Autodesk Fusion 360 part; units mm, degrees
note: some values were not read from the file. Chosen so that the rebuilt part matches the saved one: which bodies a step acts on. Set by a fixed rule: which sketch regions a step uses.
(part 2 of 2)
sketch "Sketch2" plane through (0, 0, 0) normal (0, 0, 1) x (1, 0, 0)
  line L0 (-3.5359, -0.6458) -> (-3.2779, -0.6913)
  line L1 (2.8438, -1.7707) -> (3.1017, -1.8162)
  arc A0 (3.1017, -1.8162) -> (3.681, -1.4106) centre (3.1886, -1.3238) ccw
  line L2 (3.681, -1.4106) -> (3.9414, 0.0666)
  arc A1 (3.9414, 0.0666) -> (3.5359, 0.6458) centre (3.449, 0.1534) ccw
  line L3 (3.5359, 0.6458) -> (3.2779, 0.6913)
  line L4 (-2.8438, 1.7707) -> (-3.1017, 1.8162)
  arc A2 (-3.1017, 1.8162) -> (-3.681, 1.4106) centre (-3.1886, 1.3238) ccw
  line L5 (-3.681, 1.4106) -> (-3.9414, -0.0666)
  arc A3 (-3.9414, -0.0666) -> (-3.5359, -0.6458) centre (-3.449, -0.1534) ccw
  line L6 (-1.7994, 9.2023) -> (-1.5414, 9.1568)
  line L7 (4.5803, 8.0774) -> (4.8382, 8.0319)
  arc A4 (4.8382, 8.0319) -> (5.4175, 8.4375) centre (4.925, 8.5243) ccw
  line L8 (5.4175, 8.4375) -> (5.6779, 9.9147)
  arc A5 (5.6779, 9.9147) -> (5.2723, 10.4939) centre (5.1855, 10.0015) ccw
  line L9 (5.2723, 10.4939) -> (5.0144, 10.5394)
  line L10 (-1.1073, 11.6188) -> (-1.3653, 11.6643)
  arc A6 (-1.3653, 11.6643) -> (-1.9445, 11.2587) centre (-1.4521, 11.1719) ccw
  line L11 (-1.9445, 11.2587) -> (-2.205, 9.7815)
  arc A7 (-2.205, 9.7815) -> (-1.7994, 9.2023) centre (-1.7126, 9.6947) ccw
  line L12 (-0.0629, 19.0503) -> (0.1951, 19.0049)
  line L13 (6.3167, 17.9254) -> (6.5747, 17.88)
  arc A8 (6.5747, 17.88) -> (7.1539, 18.2855) centre (6.6615, 18.3724) ccw
  line L14 (7.1539, 18.2855) -> (7.4144, 19.7627)
  arc A9 (7.4144, 19.7627) -> (7.0088, 20.342) centre (6.922, 19.8496) ccw
  line L15 (7.0088, 20.342) -> (6.7509, 20.3875)
  line L16 (0.6292, 21.4669) -> (0.3712, 21.5124)
  arc A10 (0.3712, 21.5124) -> (-0.208, 21.1068) centre (0.2844, 21.02) ccw
  line L17 (-0.208, 21.1068) -> (-0.4685, 19.6296)
  arc A11 (-0.4685, 19.6296) -> (-0.0629, 19.0503) centre (0.0239, 19.5427) ccw
  line L18 (1.6736, 28.8984) -> (1.9315, 28.8529)
  line L19 (8.0532, 27.7735) -> (8.3112, 27.728)
  arc A12 (8.3112, 27.728) -> (8.8904, 28.1336) centre (8.398, 28.2204) ccw
  line L20 (8.8904, 28.1336) -> (9.1509, 29.6108)
  arc A13 (9.1509, 29.6108) -> (8.7453, 30.19) centre (8.6585, 29.6976) ccw
  line L21 (8.7453, 30.19) -> (8.4873, 30.2355)
  line L22 (2.3657, 31.315) -> (2.1077, 31.3604)
  arc A14 (2.1077, 31.3604) -> (1.5285, 30.9549) centre (2.0209, 30.868) ccw
  line L23 (1.5285, 30.9549) -> (1.268, 29.4776)
  arc A15 (1.268, 29.4776) -> (1.6736, 28.8984) centre (1.7604, 29.3908) ccw
  line L24 (6.3122, -2.3823) -> (6.5702, -2.4278)
  line L25 (12.6919, -3.5072) -> (12.9498, -3.5527)
  arc A16 (12.9498, -3.5527) -> (13.529, -3.1471) centre (13.0366, -3.0603) ccw
  line L26 (13.529, -3.1471) -> (13.7895, -1.6699)
  arc A17 (13.7895, -1.6699) -> (13.3839, -1.0907) centre (13.2971, -1.5831) ccw
  line L27 (13.3839, -1.0907) -> (13.126, -1.0452)
  line L28 (7.0043, 0.0342) -> (6.7463, 0.0797)
  arc A18 (6.7463, 0.0797) -> (6.1671, -0.3259) centre (6.6595, -0.4127) ccw
  line L29 (6.1671, -0.3259) -> (5.9066, -1.8031)
  arc A19 (5.9066, -1.8031) -> (6.3122, -2.3823) centre (6.399, -1.8899) ccw
  line L30 (8.0487, 7.4658) -> (8.3067, 7.4203)
  line L31 (14.4283, 6.3409) -> (14.6863, 6.2954)
  arc A20 (14.6863, 6.2954) -> (15.2655, 6.701) centre (14.7731, 6.7878) ccw
  line L32 (15.2655, 6.701) -> (15.526, 8.1782)
  arc A21 (15.526, 8.1782) -> (15.1204, 8.7574) centre (15.0336, 8.265) ccw
  line L33 (15.1204, 8.7574) -> (14.8625, 8.8029)
  line L34 (8.7408, 9.8823) -> (8.4828, 9.9278)
  arc A22 (8.4828, 9.9278) -> (7.9036, 9.5222) centre (8.396, 9.4354) ccw
  line L35 (7.9036, 9.5222) -> (7.6431, 8.045)
  arc A23 (7.6431, 8.045) -> (8.0487, 7.4658) centre (8.1355, 7.9582) ccw
  line L36 (9.7852, 17.3139) -> (10.0431, 17.2684)
  line L37 (16.1648, 16.189) -> (16.4228, 16.1435)
  arc A24 (16.4228, 16.1435) -> (17.002, 16.549) centre (16.5096, 16.6359) ccw
  line L38 (17.002, 16.549) -> (17.2625, 18.0263)
  arc A25 (17.2625, 18.0263) -> (16.8569, 18.6055) centre (16.7701, 18.1131) ccw
  line L39 (16.8569, 18.6055) -> (16.5989, 18.651)
  line L40 (10.4773, 19.7304) -> (10.2193, 19.7759)
  arc A26 (10.2193, 19.7759) -> (9.6401, 19.3703) centre (10.1325, 19.2835) ccw
  line L41 (9.6401, 19.3703) -> (9.3796, 17.8931)
  arc A27 (9.3796, 17.8931) -> (9.7852, 17.3139) centre (9.872, 17.8063) ccw
  line L42 (11.5217, 27.1619) -> (11.7796, 27.1164)
  line L43 (17.9013, 26.037) -> (18.1593, 25.9915)
  arc A28 (18.1593, 25.9915) -> (18.7385, 26.3971) centre (18.2461, 26.484) ccw
  line L44 (18.7385, 26.3971) -> (18.999, 27.8743)
  arc A29 (18.999, 27.8743) -> (18.5934, 28.4536) centre (18.5066, 27.9612) ccw
  line L45 (18.5934, 28.4536) -> (18.3354, 28.4991)
  line L46 (12.2137, 29.5785) -> (11.9558, 29.624)
  arc A30 (11.9558, 29.624) -> (11.3766, 29.2184) centre (11.869, 29.1316) ccw
  line L47 (11.3766, 29.2184) -> (11.1161, 27.7412)
  arc A31 (11.1161, 27.7412) -> (11.5217, 27.1619) centre (11.6085, 27.6543) ccw
  line L48 (16.1603, -4.1188) -> (16.4183, -4.1643)
  line L49 (22.5399, -5.2437) -> (22.7979, -5.2892)
  arc A32 (22.7979, -5.2892) -> (23.3771, -4.8836) centre (22.8847, -4.7968) ccw
  line L50 (23.3771, -4.8836) -> (23.6376, -3.4064)
  arc A33 (23.6376, -3.4064) -> (23.232, -2.8271) centre (23.1452, -3.3196) ccw
  line L51 (23.232, -2.8271) -> (22.9741, -2.7817)
  line L52 (16.8524, -1.7022) -> (16.5944, -1.6568)
  arc A34 (16.5944, -1.6568) -> (16.0152, -2.0623) centre (16.5076, -2.1492) ccw
  line L53 (16.0152, -2.0623) -> (15.7547, -3.5396)
  arc A35 (15.7547, -3.5396) -> (16.1603, -4.1188) centre (16.2471, -3.6264) ccw
  line L54 (17.8968, 5.7293) -> (18.1547, 5.6838)
  line L55 (24.2764, 4.6044) -> (24.5344, 4.5589)
  arc A36 (24.5344, 4.5589) -> (25.1136, 4.9645) centre (24.6212, 5.0513) ccw
  line L56 (25.1136, 4.9645) -> (25.3741, 6.4417)
  arc A37 (25.3741, 6.4417) -> (24.9685, 7.0209) centre (24.8817, 6.5285) ccw
  line L57 (24.9685, 7.0209) -> (24.7105, 7.0664)
  line L58 (18.5889, 8.1458) -> (18.3309, 8.1913)
  arc A38 (18.3309, 8.1913) -> (17.7517, 7.7857) centre (18.2441, 7.6989) ccw
  line L59 (17.7517, 7.7857) -> (17.4912, 6.3085)
  arc A39 (17.4912, 6.3085) -> (17.8968, 5.7293) centre (17.9836, 6.2217) ccw
  line L60 (19.6333, 15.5774) -> (19.8912, 15.5319)
  line L61 (26.0129, 14.4525) -> (26.2709, 14.407)
  arc A40 (26.2709, 14.407) -> (26.8501, 14.8126) centre (26.3577, 14.8994) ccw
  line L62 (26.8501, 14.8126) -> (27.1106, 16.2898)
  arc A41 (27.1106, 16.2898) -> (26.705, 16.869) centre (26.6182, 16.3766) ccw
  line L63 (26.705, 16.869) -> (26.447, 16.9145)
  line L64 (20.3253, 17.9939) -> (20.0674, 18.0394)
  arc A42 (20.0674, 18.0394) -> (19.4881, 17.6338) centre (19.9806, 17.547) ccw
  line L65 (19.4881, 17.6338) -> (19.2277, 16.1566)
  arc A43 (19.2277, 16.1566) -> (19.6333, 15.5774) centre (19.7201, 16.0698) ccw
  line L66 (21.3697, 25.4255) -> (21.6277, 25.38)
  line L67 (27.7494, 24.3006) -> (28.0073, 24.2551)
  arc A44 (28.0073, 24.2551) -> (28.5866, 24.6606) centre (28.0942, 24.7475) ccw
  line L68 (28.5866, 24.6606) -> (28.847, 26.1379)
  arc A45 (28.847, 26.1379) -> (28.4415, 26.7171) centre (28.3546, 26.2247) ccw
  line L69 (28.4415, 26.7171) -> (28.1835, 26.7626)
  line L70 (22.0618, 27.842) -> (21.8039, 27.8875)
  arc A46 (21.8039, 27.8875) -> (21.2246, 27.4819) centre (21.717, 27.3951) ccw
  line L71 (21.2246, 27.4819) -> (20.9642, 26.0047)
  arc A47 (20.9642, 26.0047) -> (21.3697, 25.4255) centre (21.4566, 25.9179) ccw
  line L72 (26.0084, -5.8553) -> (26.2663, -5.9007)
  line L73 (32.388, -6.9802) -> (32.646, -7.0256)
  arc A48 (32.646, -7.0256) -> (33.2252, -6.6201) centre (32.7328, -6.5332) ccw
  line L74 (33.2252, -6.6201) -> (33.4857, -5.1429)
  arc A49 (33.4857, -5.1429) -> (33.0801, -4.5636) centre (32.9933, -5.056) ccw
  line L75 (33.0801, -4.5636) -> (32.8221, -4.5181)
  line L76 (26.7005, -3.4387) -> (26.4425, -3.3932)
  arc A50 (26.4425, -3.3932) -> (25.8633, -3.7988) centre (26.3557, -3.8856) ccw
  line L77 (25.8633, -3.7988) -> (25.6028, -5.276)
  arc A51 (25.6028, -5.276) -> (26.0084, -5.8553) centre (26.0952, -5.3629) ccw
  line L78 (27.7449, 3.9928) -> (28.0028, 3.9473)
  line L79 (34.1245, 2.8679) -> (34.3825, 2.8224)
  arc A52 (34.3825, 2.8224) -> (34.9617, 3.228) centre (34.4693, 3.3148) ccw
  line L80 (34.9617, 3.228) -> (35.2222, 4.7052)
  arc A53 (35.2222, 4.7052) -> (34.8166, 5.2844) centre (34.7298, 4.792) ccw
  line L81 (34.8166, 5.2844) -> (34.5586, 5.3299)
  line L82 (28.4369, 6.4093) -> (28.179, 6.4548)
  arc A54 (28.179, 6.4548) -> (27.5997, 6.0493) centre (28.0921, 5.9624) ccw
  line L83 (27.5997, 6.0493) -> (27.3393, 4.572)
  arc A55 (27.3393, 4.572) -> (27.7449, 3.9928) centre (27.8317, 4.4852) ccw
  line L84 (29.4813, 13.8409) -> (29.7393, 13.7954)
  line L85 (35.861, 12.716) -> (36.1189, 12.6705)
  arc A56 (36.1189, 12.6705) -> (36.6982, 13.0761) centre (36.2058, 13.1629) ccw
  line L86 (36.6982, 13.0761) -> (36.9586, 14.5533)
  arc A57 (36.9586, 14.5533) -> (36.5531, 15.1325) centre (36.4662, 14.6401) ccw
  line L87 (36.5531, 15.1325) -> (36.2951, 15.178)
  line L88 (30.1734, 16.2574) -> (29.9155, 16.3029)
  arc A58 (29.9155, 16.3029) -> (29.3362, 15.8973) centre (29.8286, 15.8105) ccw
  line L89 (29.3362, 15.8973) -> (29.0758, 14.4201)
  arc A59 (29.0758, 14.4201) -> (29.4813, 13.8409) centre (29.5682, 14.3333) ccw
  line L90 (31.2178, 23.689) -> (31.4758, 23.6435)
  line L91 (37.5975, 22.5641) -> (37.8554, 22.5186)
  arc A60 (37.8554, 22.5186) -> (38.4346, 22.9242) centre (37.9422, 23.011) ccw
  line L92 (38.4346, 22.9242) -> (38.6951, 24.4014)
  arc A61 (38.6951, 24.4014) -> (38.2895, 24.9806) centre (38.2027, 24.4882) ccw
  line L93 (38.2895, 24.9806) -> (38.0316, 25.0261)
  line L94 (31.9099, 26.1055) -> (31.6519, 26.151)
  arc A62 (31.6519, 26.151) -> (31.0727, 25.7454) centre (31.5651, 25.6586) ccw
  line L95 (31.0727, 25.7454) -> (30.8122, 24.2682)
  arc A63 (30.8122, 24.2682) -> (31.2178, 23.689) centre (31.3046, 24.1814) ccw
  line L96 (35.8564, -7.5917) -> (36.1144, -7.6372)
  line L97 (42.2361, -8.7166) -> (42.4941, -8.7621)
  arc A64 (42.4941, -8.7621) -> (43.0733, -8.3566) centre (42.5809, -8.2697) ccw
  line L98 (43.0733, -8.3566) -> (43.3338, -6.8793)
  arc A65 (43.3338, -6.8793) -> (42.9282, -6.3001) centre (42.8413, -6.7925) ccw
  line L99 (42.9282, -6.3001) -> (42.6702, -6.2546)
  line L100 (36.5485, -5.1752) -> (36.2906, -5.1297)
  arc A66 (36.2906, -5.1297) -> (35.7113, -5.5353) centre (36.2037, -5.6221) ccw
  line L101 (35.7113, -5.5353) -> (35.4509, -7.0125)
  arc A67 (35.4509, -7.0125) -> (35.8564, -7.5917) centre (35.9433, -7.0993) ccw
  line L102 (37.5929, 2.2563) -> (37.8509, 2.2108)
  line L103 (43.9726, 1.1314) -> (44.2305, 1.0859)
  arc A68 (44.2305, 1.0859) -> (44.8098, 1.4915) centre (44.3174, 1.5784) ccw
  line L104 (44.8098, 1.4915) -> (45.0702, 2.9687)
  arc A69 (45.0702, 2.9687) -> (44.6647, 3.548) centre (44.5778, 3.0556) ccw
  line L105 (44.6647, 3.548) -> (44.4067, 3.5935)
  line L106 (38.285, 4.6729) -> (38.0271, 4.7184)
  arc A70 (38.0271, 4.7184) -> (37.4478, 4.3128) centre (37.9402, 4.226) ccw
  line L107 (37.4478, 4.3128) -> (37.1873, 2.8356)
  arc A71 (37.1873, 2.8356) -> (37.5929, 2.2563) centre (37.6798, 2.7487) ccw
  line L108 (39.3294, 12.1044) -> (39.5874, 12.0589)
  line L109 (45.709, 10.9795) -> (45.967, 10.934)
  arc A72 (45.967, 10.934) -> (46.5462, 11.3396) centre (46.0538, 11.4264) ccw
  line L110 (46.5462, 11.3396) -> (46.8067, 12.8168)
  arc A73 (46.8067, 12.8168) -> (46.4011, 13.396) centre (46.3143, 12.9036) ccw
  line L111 (46.4011, 13.396) -> (46.1432, 13.4415)
  line L112 (40.0215, 14.5209) -> (39.7635, 14.5664)
  arc A74 (39.7635, 14.5664) -> (39.1843, 14.1609) centre (39.6767, 14.074) ccw
  line L113 (39.1843, 14.1609) -> (38.9238, 12.6836)
  arc A75 (38.9238, 12.6836) -> (39.3294, 12.1044) centre (39.4162, 12.5968) ccw
  line L114 (41.0659, 21.9525) -> (41.3239, 21.907)
  line L115 (47.4455, 20.8276) -> (47.7035, 20.7821)
  arc A76 (47.7035, 20.7821) -> (48.2827, 21.1877) centre (47.7903, 21.2745) ccw
  line L116 (48.2827, 21.1877) -> (48.5432, 22.6649)
  arc A77 (48.5432, 22.6649) -> (48.1376, 23.2441) centre (48.0508, 22.7517) ccw
  line L117 (48.1376, 23.2441) -> (47.8797, 23.2896)
  line L118 (41.758, 24.369) -> (41.5, 24.4145)
  arc A78 (41.5, 24.4145) -> (40.9208, 24.0089) centre (41.4132, 23.9221) ccw
  line L119 (40.9208, 24.0089) -> (40.6603, 22.5317)
  arc A79 (40.6603, 22.5317) -> (41.0659, 21.9525) centre (41.1527, 22.4449) ccw
  line L120 (101.6288, -1.8162) -> (101.8868, -1.7707)
  line L121 (108.0084, -0.6913) -> (108.2664, -0.6458)
  arc A80 (108.2664, -0.6458) -> (108.672, -0.0666) centre (108.1796, -0.1534) ccw
  line L122 (108.672, -0.0666) -> (108.4115, 1.4106)
  arc A81 (108.4115, 1.4106) -> (107.8323, 1.8162) centre (107.9191, 1.3238) ccw
  line L123 (107.8323, 1.8162) -> (107.5743, 1.7707)
  line L124 (101.4527, 0.6913) -> (101.1947, 0.6458)
  arc A82 (101.1947, 0.6458) -> (100.7891, 0.0666) centre (101.2815, 0.1534) ccw
  line L125 (100.7891, 0.0666) -> (101.0496, -1.4106)
  arc A83 (101.0496, -1.4106) -> (101.6288, -1.8162) centre (101.542, -1.3238) ccw
  line L126 (99.8923, 8.0319) -> (100.1503, 8.0774)
  line L127 (106.272, 9.1568) -> (106.5299, 9.2023)
  arc A84 (106.5299, 9.2023) -> (106.9355, 9.7815) centre (106.4431, 9.6947) ccw
  line L128 (106.9355, 9.7815) -> (106.675, 11.2587)
  arc A85 (106.675, 11.2587) -> (106.0958, 11.6643) centre (106.1826, 11.1719) ccw
  line L129 (106.0958, 11.6643) -> (105.8378, 11.6188)
  line L130 (99.7162, 10.5394) -> (99.4582, 10.4939)
  arc A86 (99.4582, 10.4939) -> (99.0526, 9.9147) centre (99.545, 10.0015) ccw
  line L131 (99.0526, 9.9147) -> (99.3131, 8.4375)
  arc A87 (99.3131, 8.4375) -> (99.8923, 8.0319) centre (99.8055, 8.5243) ccw
  line L132 (98.1558, 17.88) -> (98.4138, 17.9254)
  line L133 (104.5355, 19.0049) -> (104.7934, 19.0503)
  arc A88 (104.7934, 19.0503) -> (105.199, 19.6296) centre (104.7066, 19.5427) ccw
  line L134 (105.199, 19.6296) -> (104.9386, 21.1068)
  arc A89 (104.9386, 21.1068) -> (104.3593, 21.5124) centre (104.4461, 21.02) ccw
  line L135 (104.3593, 21.5124) -> (104.1014, 21.4669)
  line L136 (97.9797, 20.3875) -> (97.7217, 20.342)
  arc A90 (97.7217, 20.342) -> (97.3161, 19.7627) centre (97.8085, 19.8496) ccw
  line L137 (97.3161, 19.7627) -> (97.5766, 18.2855)
  arc A91 (97.5766, 18.2855) -> (98.1558, 17.88) centre (98.069, 18.3724) ccw
  line L138 (96.4194, 27.728) -> (96.6773, 27.7735)
  line L139 (102.799, 28.8529) -> (103.057, 28.8984)
  arc A92 (103.057, 28.8984) -> (103.4625, 29.4776) centre (102.9701, 29.3908) ccw
  line L140 (103.4625, 29.4776) -> (103.2021, 30.9549)
  arc A93 (103.2021, 30.9549) -> (102.6228, 31.3604) centre (102.7097, 30.868) ccw
  line L141 (102.6228, 31.3604) -> (102.3649, 31.315)
  line L142 (96.2432, 30.2355) -> (95.9852, 30.19)
  arc A94 (95.9852, 30.19) -> (95.5797, 29.6108) centre (96.0721, 29.6976) ccw
  line L143 (95.5797, 29.6108) -> (95.8401, 28.1336)
  arc A95 (95.8401, 28.1336) -> (96.4194, 27.728) centre (96.3325, 28.2204) ccw
  line L144 (91.7807, -3.5527) -> (92.0387, -3.5072)
  line L145 (98.1604, -2.4278) -> (98.4183, -2.3823)
  arc A96 (98.4183, -2.3823) -> (98.8239, -1.8031) centre (98.3315, -1.8899) ccw
  line L146 (98.8239, -1.8031) -> (98.5634, -0.3259)
  arc A97 (98.5634, -0.3259) -> (97.9842, 0.0797) centre (98.071, -0.4127) ccw
  line L147 (97.9842, 0.0797) -> (97.7262, 0.0342)
  line L148 (91.6046, -1.0452) -> (91.3466, -1.0907)
  arc A98 (91.3466, -1.0907) -> (90.941, -1.6699) centre (91.4334, -1.5831) ccw
  line L149 (90.941, -1.6699) -> (91.2015, -3.1471)
  arc A99 (91.2015, -3.1471) -> (91.7807, -3.5527) centre (91.6939, -3.0603) ccw
  line L150 (90.0442, 6.2954) -> (90.3022, 6.3409)
  line L151 (96.4239, 7.4203) -> (96.6819, 7.4658)
  arc A100 (96.6819, 7.4658) -> (97.0874, 8.045) centre (96.595, 7.9582) ccw
  line L152 (97.0874, 8.045) -> (96.827, 9.5222)
  arc A101 (96.827, 9.5222) -> (96.2477, 9.9278) centre (96.3346, 9.4354) ccw
  line L153 (96.2477, 9.9278) -> (95.9898, 9.8823)
  line L154 (89.8681, 8.8029) -> (89.6101, 8.7574)
  arc A102 (89.6101, 8.7574) -> (89.2045, 8.1782) centre (89.6969, 8.265) ccw
  line L155 (89.2045, 8.1782) -> (89.465, 6.701)
  arc A103 (89.465, 6.701) -> (90.0442, 6.2954) centre (89.9574, 6.7878) ccw
  line L156 (88.3078, 16.1435) -> (88.5657, 16.189)
  line L157 (94.6874, 17.2684) -> (94.9454, 17.3139)
  arc A104 (94.9454, 17.3139) -> (95.3509, 17.8931) centre (94.8585, 17.8063) ccw
  line L158 (95.3509, 17.8931) -> (95.0905, 19.3703)
  arc A105 (95.0905, 19.3703) -> (94.5112, 19.7759) centre (94.5981, 19.2835) ccw
  line L159 (94.5112, 19.7759) -> (94.2533, 19.7304)
  line L160 (88.1316, 18.651) -> (87.8736, 18.6055)
  arc A106 (87.8736, 18.6055) -> (87.4681, 18.0263) centre (87.9605, 18.1131) ccw
  line L161 (87.4681, 18.0263) -> (87.7285, 16.549)
  arc A107 (87.7285, 16.549) -> (88.3078, 16.1435) centre (88.2209, 16.6359) ccw
  line L162 (86.5713, 25.9915) -> (86.8292, 26.037)
  line L163 (92.9509, 27.1164) -> (93.2089, 27.1619)
  arc A108 (93.2089, 27.1619) -> (93.6145, 27.7412) centre (93.1221, 27.6543) ccw
  line L164 (93.6145, 27.7412) -> (93.354, 29.2184)
  arc A109 (93.354, 29.2184) -> (92.7748, 29.624) centre (92.8616, 29.1316) ccw
  line L165 (92.7748, 29.624) -> (92.5168, 29.5785)
  line L166 (86.3951, 28.4991) -> (86.1372, 28.4536)
  arc A110 (86.1372, 28.4536) -> (85.7316, 27.8743) centre (86.224, 27.9612) ccw
  line L167 (85.7316, 27.8743) -> (85.9921, 26.3971)
  arc A111 (85.9921, 26.3971) -> (86.5713, 25.9915) centre (86.4845, 26.484) ccw
  line L168 (81.9327, -5.2892) -> (82.1906, -5.2437)
  line L169 (88.3123, -4.1643) -> (88.5703, -4.1188)
  arc A112 (88.5703, -4.1188) -> (88.9758, -3.5396) centre (88.4834, -3.6264) ccw
  line L170 (88.9758, -3.5396) -> (88.7154, -2.0623)
  arc A113 (88.7154, -2.0623) -> (88.1361, -1.6568) centre (88.223, -2.1492) ccw
  line L171 (88.1361, -1.6568) -> (87.8782, -1.7022)
  line L172 (81.7565, -2.7817) -> (81.4985, -2.8271)
  arc A114 (81.4985, -2.8271) -> (81.093, -3.4064) centre (81.5854, -3.3196) ccw
  line L173 (81.093, -3.4064) -> (81.3534, -4.8836)
  arc A115 (81.3534, -4.8836) -> (81.9327, -5.2892) centre (81.8458, -4.7968) ccw
  line L174 (80.1962, 4.5589) -> (80.4541, 4.6044)
  line L175 (86.5758, 5.6838) -> (86.8338, 5.7293)
  arc A116 (86.8338, 5.7293) -> (87.2394, 6.3085) centre (86.7469, 6.2217) ccw
  line L176 (87.2394, 6.3085) -> (86.9789, 7.7857)
  arc A117 (86.9789, 7.7857) -> (86.3997, 8.1913) centre (86.4865, 7.6989) ccw
  line L177 (86.3997, 8.1913) -> (86.1417, 8.1458)
  line L178 (80.02, 7.0664) -> (79.762, 7.0209)
  arc A118 (79.762, 7.0209) -> (79.3565, 6.4417) centre (79.8489, 6.5285) ccw
  line L179 (79.3565, 6.4417) -> (79.6169, 4.9645)
  arc A119 (79.6169, 4.9645) -> (80.1962, 4.5589) centre (80.1093, 5.0513) ccw
  line L180 (78.4597, 14.407) -> (78.7177, 14.4525)
  line L181 (84.8393, 15.5319) -> (85.0973, 15.5774)
  arc A120 (85.0973, 15.5774) -> (85.5029, 16.1566) centre (85.0105, 16.0698) ccw
  line L182 (85.5029, 16.1566) -> (85.2424, 17.6338)
  arc A121 (85.2424, 17.6338) -> (84.6632, 18.0394) centre (84.75, 17.547) ccw
  line L183 (84.6632, 18.0394) -> (84.4052, 17.9939)
  line L184 (78.2835, 16.9145) -> (78.0256, 16.869)
  arc A122 (78.0256, 16.869) -> (77.62, 16.2898) centre (78.1124, 16.3766) ccw
  line L185 (77.62, 16.2898) -> (77.8805, 14.8126)
  arc A123 (77.8805, 14.8126) -> (78.4597, 14.407) centre (78.3729, 14.8994) ccw
  line L186 (76.7232, 24.2551) -> (76.9812, 24.3006)
  line L187 (83.1028, 25.38) -> (83.3608, 25.4255)
  arc A124 (83.3608, 25.4255) -> (83.7664, 26.0047) centre (83.274, 25.9179) ccw
  line L188 (83.7664, 26.0047) -> (83.5059, 27.4819)
  arc A125 (83.5059, 27.4819) -> (82.9267, 27.8875) centre (83.0135, 27.3951) ccw
  line L189 (82.9267, 27.8875) -> (82.6687, 27.842)
  line L190 (76.5471, 26.7626) -> (76.2891, 26.7171)
  arc A126 (76.2891, 26.7171) -> (75.8835, 26.1379) centre (76.3759, 26.2247) ccw
  line L191 (75.8835, 26.1379) -> (76.144, 24.6606)
  arc A127 (76.144, 24.6606) -> (76.7232, 24.2551) centre (76.6364, 24.7475) ccw
  line L192 (72.0846, -7.0256) -> (72.3425, -6.9802)
  line L193 (78.4642, -5.9007) -> (78.7222, -5.8553)
  arc A128 (78.7222, -5.8553) -> (79.1278, -5.276) centre (78.6354, -5.3629) ccw
  line L194 (79.1278, -5.276) -> (78.8673, -3.7988)
  arc A129 (78.8673, -3.7988) -> (78.2881, -3.3932) centre (78.3749, -3.8856) ccw
  line L195 (78.2881, -3.3932) -> (78.0301, -3.4387)
  line L196 (71.9084, -4.5181) -> (71.6505, -4.5636)
  arc A130 (71.6505, -4.5636) -> (71.2449, -5.1429) centre (71.7373, -5.056) ccw
  line L197 (71.2449, -5.1429) -> (71.5053, -6.6201)
  arc A131 (71.5053, -6.6201) -> (72.0846, -7.0256) centre (71.9977, -6.5332) ccw
  line L198 (70.3481, 2.8224) -> (70.6061, 2.8679)
  line L199 (76.7277, 3.9473) -> (76.9857, 3.9928)
  arc A132 (76.9857, 3.9928) -> (77.3913, 4.572) centre (76.8989, 4.4852) ccw
  line L200 (77.3913, 4.572) -> (77.1308, 6.0493)
  arc A133 (77.1308, 6.0493) -> (76.5516, 6.4548) centre (76.6384, 5.9624) ccw
  line L201 (76.5516, 6.4548) -> (76.2936, 6.4093)
  line L202 (70.1719, 5.3299) -> (69.914, 5.2844)
  arc A134 (69.914, 5.2844) -> (69.5084, 4.7052) centre (70.0008, 4.792) ccw
  line L203 (69.5084, 4.7052) -> (69.7689, 3.228)
  arc A135 (69.7689, 3.228) -> (70.3481, 2.8224) centre (70.2613, 3.3148) ccw
  line L204 (68.6116, 12.6705) -> (68.8696, 12.716)
  line L205 (74.9912, 13.7954) -> (75.2492, 13.8409)
  arc A136 (75.2492, 13.8409) -> (75.6548, 14.4201) centre (75.1624, 14.3333) ccw
  line L206 (75.6548, 14.4201) -> (75.3943, 15.8973)
  arc A137 (75.3943, 15.8973) -> (74.8151, 16.3029) centre (74.9019, 15.8105) ccw
  line L207 (74.8151, 16.3029) -> (74.5571, 16.2574)
  line L208 (68.4355, 15.178) -> (68.1775, 15.1325)
  arc A138 (68.1775, 15.1325) -> (67.7719, 14.5533) centre (68.2643, 14.6401) ccw
  line L209 (67.7719, 14.5533) -> (68.0324, 13.0761)
  arc A139 (68.0324, 13.0761) -> (68.6116, 12.6705) centre (68.5248, 13.1629) ccw
  line L210 (66.8751, 22.5186) -> (67.1331, 22.5641)
  line L211 (73.2548, 23.6435) -> (73.5127, 23.689)
  arc A140 (73.5127, 23.689) -> (73.9183, 24.2682) centre (73.4259, 24.1814) ccw
  line L212 (73.9183, 24.2682) -> (73.6578, 25.7454)
  arc A141 (73.6578, 25.7454) -> (73.0786, 26.151) centre (73.1654, 25.6586) ccw
  line L213 (73.0786, 26.151) -> (72.8206, 26.1055)
  line L214 (66.699, 25.0261) -> (66.441, 24.9806)
  arc A142 (66.441, 24.9806) -> (66.0354, 24.4014) centre (66.5278, 24.4882) ccw
  line L215 (66.0354, 24.4014) -> (66.2959, 22.9242)
  arc A143 (66.2959, 22.9242) -> (66.8751, 22.5186) centre (66.7883, 23.011) ccw
  line L216 (62.2365, -8.7621) -> (62.4945, -8.7166)
  line L217 (68.6161, -7.6372) -> (68.8741, -7.5917)
  arc A144 (68.8741, -7.5917) -> (69.2797, -7.0125) centre (68.7873, -7.0993) ccw
  line L218 (69.2797, -7.0125) -> (69.0192, -5.5353)
  arc A145 (69.0192, -5.5353) -> (68.44, -5.1297) centre (68.5268, -5.6221) ccw
  line L219 (68.44, -5.1297) -> (68.182, -5.1752)
  line L220 (62.0603, -6.2546) -> (61.8024, -6.3001)
  arc A146 (61.8024, -6.3001) -> (61.3968, -6.8793) centre (61.8892, -6.7925) ccw
  line L221 (61.3968, -6.8793) -> (61.6573, -8.3566)
  arc A147 (61.6573, -8.3566) -> (62.2365, -8.7621) centre (62.1497, -8.2697) ccw
  line L222 (60.5, 1.0859) -> (60.758, 1.1314)
  line L223 (66.8797, 2.2108) -> (67.1376, 2.2563)
  arc A148 (67.1376, 2.2563) -> (67.5432, 2.8356) centre (67.0508, 2.7487) ccw
  line L224 (67.5432, 2.8356) -> (67.2827, 4.3128)
  arc A149 (67.2827, 4.3128) -> (66.7035, 4.7184) centre (66.7903, 4.226) ccw
  line L225 (66.7035, 4.7184) -> (66.4455, 4.6729)
  line L226 (60.3239, 3.5935) -> (60.0659, 3.548)
  arc A150 (60.0659, 3.548) -> (59.6603, 2.9687) centre (60.1527, 3.0556) ccw
  line L227 (59.6603, 2.9687) -> (59.9208, 1.4915)
  arc A151 (59.9208, 1.4915) -> (60.5, 1.0859) centre (60.4132, 1.5784) ccw
  line L228 (58.7635, 10.934) -> (59.0215, 10.9795)
  line L229 (65.1432, 12.0589) -> (65.4011, 12.1044)
  arc A152 (65.4011, 12.1044) -> (65.8067, 12.6836) centre (65.3143, 12.5968) ccw
  line L230 (65.8067, 12.6836) -> (65.5462, 14.1609)
  arc A153 (65.5462, 14.1609) -> (64.967, 14.5664) centre (65.0538, 14.074) ccw
  line L231 (64.967, 14.5664) -> (64.709, 14.5209)
  line L232 (58.5874, 13.4415) -> (58.3294, 13.396)
  arc A154 (58.3294, 13.396) -> (57.9238, 12.8168) centre (58.4162, 12.9036) ccw
  line L233 (57.9238, 12.8168) -> (58.1843, 11.3396)
  arc A155 (58.1843, 11.3396) -> (58.7635, 10.934) centre (58.6767, 11.4264) ccw
  line L234 (57.0271, 20.7821) -> (57.285, 20.8276)
  line L235 (63.4067, 21.907) -> (63.6647, 21.9525)
  arc A156 (63.6647, 21.9525) -> (64.0702, 22.5317) centre (63.5778, 22.4449) ccw
  line L236 (64.0702, 22.5317) -> (63.8098, 24.0089)
  arc A157 (63.8098, 24.0089) -> (63.2305, 24.4145) centre (63.3174, 23.9221) ccw
  line L237 (63.2305, 24.4145) -> (62.9726, 24.369)
  line L238 (56.8509, 23.2896) -> (56.5929, 23.2441)
  arc A158 (56.5929, 23.2441) -> (56.1873, 22.6649) centre (56.6798, 22.7517) ccw
  line L239 (56.1873, 22.6649) -> (56.4478, 21.1877)
  arc A159 (56.4478, 21.1877) -> (57.0271, 20.7821) centre (56.9402, 21.2745) ccw
  arc A160 (-3.2779, -0.6913) -> (-3.2779, -0.6913) centre (0, 0) ccw
  arc A161 (-1.5414, 9.1568) -> (-1.5414, 9.1568) centre (1.7365, 9.8481) ccw
  arc A162 (0.1951, 19.0049) -> (0.1951, 19.0049) centre (3.473, 19.6962) ccw
  arc A163 (1.9315, 28.8529) -> (1.9315, 28.8529) centre (5.2094, 29.5442) ccw
  arc A164 (6.5702, -2.4278) -> (6.5702, -2.4278) centre (9.8481, -1.7365) ccw
  arc A165 (8.3067, 7.4203) -> (8.3067, 7.4203) centre (11.5846, 8.1116) ccw
  arc A166 (10.0431, 17.2684) -> (10.0431, 17.2684) centre (13.321, 17.9597) ccw
  arc A167 (11.7796, 27.1164) -> (11.7796, 27.1164) centre (15.0575, 27.8078) ccw
  arc A168 (16.4183, -4.1643) -> (16.4183, -4.1643) centre (19.6962, -3.473) ccw
  arc A169 (18.1547, 5.6838) -> (18.1547, 5.6838) centre (21.4326, 6.3751) ccw
  arc A170 (19.8912, 15.5319) -> (19.8912, 15.5319) centre (23.1691, 16.2232) ccw
  arc A171 (21.6277, 25.38) -> (21.6277, 25.38) centre (24.9056, 26.0713) ccw
  arc A172 (26.2663, -5.9007) -> (26.2663, -5.9007) centre (29.5442, -5.2094) ccw
  arc A173 (28.0028, 3.9473) -> (28.0028, 3.9473) centre (31.2807, 4.6386) ccw
  arc A174 (29.7393, 13.7954) -> (29.7393, 13.7954) centre (33.0172, 14.4867) ccw
  arc A175 (31.4758, 23.6435) -> (31.4758, 23.6435) centre (34.7537, 24.3348) ccw
  arc A176 (36.1144, -7.6372) -> (36.1144, -7.6372) centre (39.3923, -6.9459) ccw
  arc A177 (37.8509, 2.2108) -> (37.8509, 2.2108) centre (41.1288, 2.9022) ccw
  arc A178 (39.5874, 12.0589) -> (39.5874, 12.0589) centre (42.8653, 12.7502) ccw
  arc A179 (41.3239, 21.907) -> (41.3239, 21.907) centre (44.6018, 22.5983) ccw
  circle A180 centre (104.7305, 0) radius 3.35
  circle A181 centre (102.9941, 9.8481) radius 3.35
  circle A182 centre (101.2576, 19.6962) radius 3.35
  circle A183 centre (99.5211, 29.5442) radius 3.35
  circle A184 centre (94.8825, -1.7365) radius 3.35
  circle A185 centre (93.146, 8.1116) radius 3.35
  circle A186 centre (91.4095, 17.9597) radius 3.35
  circle A187 centre (89.673, 27.8078) radius 3.35
  circle A188 centre (85.0344, -3.473) radius 3.35
  circle A189 centre (83.2979, 6.3751) radius 3.35
  circle A190 centre (81.5614, 16.2232) radius 3.35
  circle A191 centre (79.8249, 26.0713) radius 3.35
  circle A192 centre (75.1863, -5.2094) radius 3.35
  circle A193 centre (73.4498, 4.6386) radius 3.35
  circle A194 centre (71.7134, 14.4867) radius 3.35
  circle A195 centre (69.9769, 24.3348) radius 3.35
  circle A196 centre (65.3382, -6.9459) radius 3.35
  circle A197 centre (63.6018, 2.9022) radius 3.35
  circle A198 centre (61.8653, 12.7502) radius 3.35
  circle A199 centre (60.1288, 22.5983) radius 3.35
  circle A200 centre (5.2094, 29.5442) radius 3.35
  circle A201 centre (15.0575, 27.8078) radius 3.35
  circle A202 centre (24.9056, 26.0713) radius 3.35
  circle A203 centre (34.7537, 24.3348) radius 3.35
  circle A204 centre (44.6018, 22.5983) radius 3.35
  circle A205 centre (42.8653, 12.7502) radius 3.35
  circle A206 centre (33.0172, 14.4867) radius 3.35
  circle A207 centre (23.1691, 16.2232) radius 3.35
  circle A208 centre (13.321, 17.9597) radius 3.35
  circle A209 centre (3.473, 19.6962) radius 3.35
  circle A210 centre (1.7365, 9.8481) radius 3.35
  circle A211 centre (11.5846, 8.1116) radius 3.35
  circle A212 centre (21.4326, 6.3751) radius 3.35
  circle A213 centre (31.2807, 4.6386) radius 3.35
  circle A214 centre (41.1288, 2.9022) radius 3.35
  circle A215 centre (39.3923, -6.9459) radius 3.35
  circle A216 centre (29.5442, -5.2094) radius 3.35
  circle A217 centre (19.6962, -3.473) radius 3.35
  circle A218 centre (9.8481, -1.7365) radius 3.35
  circle A219 centre (0, 0) radius 3.35
  constraint concentric A163 A200
  constraint coincident L19.start A200
  constraint concentric A167 A201
  constraint coincident L43.start A201
  constraint concentric A171 A202
  constraint coincident L67.start A202
  constraint concentric A175 A203
  constraint coincident L90.end A203
  constraint coincident L114.end A204
  constraint concentric A178 A205
  constraint coincident L108.end A205
  constraint coincident L84.end A206
  constraint coincident L60.end A207
  constraint coincident L36.end A208
  constraint coincident L12.end A209
  constraint coincident L6.end A210
  constraint coincident L30.end A211
  constraint coincident L54.end A212
  constraint coincident L78.end A213
  constraint coincident L102.end A214
  constraint concentric A176 A215
  constraint coincident L96.end A215
  constraint coincident L72.end A216
  constraint coincident L48.end A217
  constraint coincident L24.end A218
  constraint coincident L0.end A219
extrude "Extrude1" add sketch "Sketch1" along normal blind 2.5 contours L6 L7 L8 L9 L10 L11 A6 A7 A8 A9 A10 A11 | L12 L13 L14 L15 L16 L17 A12 A13 A14 A15 A16 A17 makes body 1
extrude "Extrude2" add sketch "Sketch1" along normal blind 5.1 contours A218 | A219 | A220 | A221 | A222 | A223 | A224 | A225 bodies 1
extrude "Extrude3" add sketch "Sketch1" along normal blind 6.7 contours L0 L1 L2 L3 L4 L5 A0 A1 A2 A3 A4 A5 bodies 1
extrude "Extrude5" add sketch "Sketch1" along normal blind 0.5 contours L18 L22 A20 L23 A21 A178 A234 | L19 A18 L20 A19 L21 A178 A234 | L24 L28 A24 L29 A25 A179 A235 | L25 A22 L26 A23 L27 A179 A235 | L30 L34 A28 L35 A29 A180 A236 | L31 A26 L32 A27 L33 A180 A236 | L36 L40 A32 L41 A33 A181 A237 | L37 A30 L38 A31 L39 A181 A237 | L42 L46 A36 L47 A37 A182 A241 | L43 A34 L44 A35 L45 A182 A241 | L48 L52 A40 L53 A41 A183 A240 | L49 A38 L50 A39 L51 A183 A240 | L54 L58 A44 L59 A45 A184 A239 | L55 A42 L56 A43 L57 A184 A239 | L60 L64 A48 L65 A49 A185 A238 | L61 A46 L62 A47 L63 A185 A238 | L66 L70 A52 L71 A53 A186 A242 | L67 A50 L68 A51 L69 A186 A242 | L72 L76 A56 L77 A57 A187 A243 | L73 A54 L74 A55 L75 A187 A243 | L78 L82 A60 L83 A61 A188 A244 | L79 A58 L80 A59 L81 A188 A244 | L84 L88 A64 L89 A65 A189 A245 | L85 A62 L86 A63 L87 A189 A245 | L90 L94 A68 L95 A69 A190 A249 | L91 A66 L92 A67 L93 A190 A249 | L96 L100 A72 L101 A73 A191 A248 | L97 A70 L98 A71 L99 A191 A248 | L102 L106 A76 L107 A77 A192 A247 | L103 A74 L104 A75 L105 A192 A247 | L108 L112 A80 L113 A81 A193 A246 | L109 A78 L110 A79 L111 A193 A246 | L114 L118 A84 L119 A85 A194 A250 | L115 A82 L116 A83 L117 A194 A250 | L120 L124 A88 L125 A89 A195 A251 | L121 A86 L122 A87 L123 A195 A251 | L126 L130 A92 L131 A93 A196 A252 | L127 A90 L128 A91 L129 A196 A252 | L132 L136 A96 L137 A97 A197 A253 | L133 A94 L134 A95 L135 A197 A253 | L138 L142 A100 L143 A101 A198 A273 | L139 A98 L140 A99 L141 A198 A273 | L144 L148 A104 L149 A105 A199 A272 | L145 A102 L146 A103 L147 A199 A272 | L150 L154 A108 L155 A109 A200 A271 | L151 A106 L152 A107 L153 A200 A271 | L156 L160 A112 L161 A113 A201 A270 | L157 A110 L158 A111 L159 A201 A270 | L162 L166 A116 L167 A117 A202 A266 | L163 A114 L164 A115 L165 A202 A266 | L168 L172 A120 L173 A121 A203 A267 | L169 A118 L170 A119 L171 A203 A267 | L174 L178 A124 L179 A125 A204 A268 | L175 A122 L176 A123 L177 A204 A268 | L180 L184 A128 L185 A129 A205 A269 | L181 A126 L182 A127 L183 A205 A269 | L186 L190 A132 L191 A133 A206 A265 | L187 A130 L188 A131 L189 A206 A265 | L192 L196 A136 L197 A137 A207 A264 | L193 A134 L194 A135 L195 A207 A264 | L198 L202 A140 L203 A141 A208 A263 | L199 A138 L200 A139 L201 A208 A263 | L204 L208 A144 L209 A145 A209 A262 | L205 A142 L206 A143 L207 A209 A262 | L210 L214 A148 L215 A149 A210 A258 | L211 A146 L212 A147 L213 A210 A258 | L216 L220 A152 L221 A153 A211 A259 | L217 A150 L218 A151 L219 A211 A259 | L222 L226 A156 L227 A157 A212 A260 | L223 A154 L224 A155 L225 A212 A260 | L228 L232 A160 L233 A161 A213 A261 | L229 A158 L230 A159 L231 A213 A261 | L234 L238 A164 L239 A165 A214 A257 | L235 A162 L236 A163 L237 A214 A257 | L240 L244 A168 L245 A169 A215 A256 | L241 A166 L242 A167 L243 A215 A256 | L246 L250 A172 L251 A173 A216 A255 | L247 A170 L248 A171 L249 A216 A255 | L252 L256 A176 L257 A177 A217 A254 | L253 A174 L254 A175 L255 A217 A254 bodies 1
extrude "Extrude7" add sketch "Sketch2" along normal blind 4 separate body contours A160 A219 | A161 A210 | A162 A209 | A163 A200 | A164 A218 | A165 A211 | A166 A208 | A167 A201 | A168 A217 | A169 A212 | A170 A207 | A171 A202 | A172 A216 | A173 A213 | A174 A206 | A175 A203 | A176 A215 | A177 A214 | A178 A205 | A179 A204 | A180 | A181 | A182 | A183 | A184 | A185 | A186 | A187 | A188 | A189 | A190 | A191 | A192 | A193 | A194 | A195 | A196 | A197 | A198 | A199 makes body 2 at (90.3426, 14.7841, 1.3333) makes body 3 at (24.7785, 6.2081, 1.3333) makes body 4 at (93.8155, -4.912, 1.3333) makes body 5 at (13.1939, -1.9035, 1.3333) makes body 6 at (83.9675, -6.6485, 1.3333) makes body 7 at (63.4621, 22.9319, 2.6667) makes body 8 at (36.3505, 14.8203, 2.6667) makes body 9 at (28.239, 26.4048, 2.6667) makes body 10 at (8.5428, 29.8778, 2.6667) makes body 11 at (16.6544, 18.2932, 2.6667) makes body 12 at (97.5656, 26.8242, 1.3333) makes body 13 at (74.1194, -8.385, 1.3333) makes body 14 at (68.0213, 21.6148, 1.3333) makes body 15 at (88.6061, 24.6322, 1.3333) makes body 16 at (64.2713, -10.1215, 1.3333) makes body 17 at (3.3458, -0.167, 1.3333) makes body 18 at (44.4621, 3.2357, 2.6667) makes body 19 at (18.3909, 28.1413, 2.6667) makes body 20 at (77.8694, 23.3513, 1.3333) makes body 21 at (42.7257, -6.6124, 2.6667) makes body 22 at (64.0183, -0.4219, 1.3333) makes body 23 at (14.9179, 8.4451, 2.6667) makes body 24 at (46.2111, 12.5832, 1.3333) makes body 25 at (34.6141, 4.9722, 2.6667) makes body 26 at (80.4945, 13.0476, 1.3333) makes body 27 at (70.6464, 11.3112, 1.3333) makes body 28 at (103.6636, -3.1756, 1.3333) makes body 29 at (100.1907, 16.5206, 1.3333) makes body 30 at (92.0791, 4.936, 1.3333) makes body 31 at (32.8901, -5.3764, 1.3333) makes body 32 at (72.3829, 1.4631, 1.3333) makes body 33 at (82.231, 3.1996, 1.3333) makes body 34 at (101.9271, 6.6725, 1.3333) makes body 35 at (47.9476, 22.4313, 1.3333) makes body 36 at (6.8188, 19.5292, 1.3333) makes body 37 at (26.5025, 16.5567, 2.6667) makes body 38 at (23.042, -3.6399, 1.3333) makes body 39 at (38.0995, 24.1678, 1.3333) makes body 40 at (60.337, 9.7692, 2.6667) makes body 41 at (5.0823, 9.6811, 1.3333)
extrude "Extrude6" add sketch "Sketch2" along normal blind 2 contours L0 L4 A2 L5 A3 A160 A219 | L1 A0 L2 A1 L3 A160 A219 | L6 L10 A6 L11 A7 A161 A210 | L7 A4 L8 A5 L9 A161 A210 | L12 L16 A10 L17 A11 A162 A209 | L13 A8 L14 A9 L15 A162 A209 | L18 L22 A14 L23 A15 A163 A200 | L19 A12 L20 A13 L21 A163 A200 | L24 L28 A18 L29 A19 A164 A218 | L25 A16 L26 A17 L27 A164 A218 | L30 L34 A22 L35 A23 A165 A211 | L31 A20 L32 A21 L33 A165 A211 | L36 L40 A26 L41 A27 A166 A208 | L37 A24 L38 A25 L39 A166 A208 | L42 L46 A30 L47 A31 A167 A201 | L43 A28 L44 A29 L45 A167 A201 | L48 L52 A34 L53 A35 A168 A217 | L49 A32 L50 A33 L51 A168 A217 | L54 L58 A38 L59 A39 A169 A212 | L55 A36 L56 A37 L57 A169 A212 | L60 L64 A42 L65 A43 A170 A207 | L61 A40 L62 A41 L63 A170 A207 | L66 L70 A46 L71 A47 A171 A202 | L67 A44 L68 A45 L69 A171 A202 | L72 L76 A50 L77 A51 A172 A216 | L73 A48 L74 A49 L75 A172 A216 | L78 L82 A54 L83 A55 A173 A213 | L79 A52 L80 A53 L81 A173 A213 | L84 L88 A58 L89 A59 A174 A206 | L85 A56 L86 A57 L87 A174 A206 | L90 L94 A62 L95 A63 A175 A203 | L91 A60 L92 A61 L93 A175 A203 | L96 L100 A66 L101 A67 A176 A215 | L97 A64 L98 A65 L99 A176 A215 | L102 L106 A70 L107 A71 A177 A214 | L103 A68 L104 A69 L105 A177 A214 | L108 L112 A74 L113 A75 A178 A205 | L109 A72 L110 A73 L111 A178 A205 | L114 L118 A78 L119 A79 A179 A204 | L115 A76 L116 A77 L117 A179 A204 | L120 L124 A82 L125 A83 A180 | L121 A80 L122 A81 L123 A180 | L126 L130 A86 L131 A87 A181 | L127 A84 L128 A85 L129 A181 | L132 L136 A90 L137 A91 A182 | L133 A88 L134 A89 L135 A182 | L138 L142 A94 L143 A95 A183 | L139 A92 L140 A93 L141 A183 | L144 L148 A98 L149 A99 A184 | L145 A96 L146 A97 L147 A184 | L150 L154 A102 L155 A103 A185 | L151 A100 L152 A101 L153 A185 | L156 L160 A106 L161 A107 A186 | L157 A104 L158 A105 L159 A186 | L162 L166 A110 L167 A111 A187 | L163 A108 L164 A109 L165 A187 | L168 L172 A114 L173 A115 A188 | L169 A112 L170 A113 L171 A188 | L174 L178 A118 L179 A119 A189 | L175 A116 L176 A117 L177 A189 | L180 L184 A122 L185 A123 A190 | L181 A120 L182 A121 L183 A190 | L186 L190 A126 L191 A127 A191 | L187 A124 L188 A125 L189 A191 | L192 L196 A130 L197 A131 A192 | L193 A128 L194 A129 L195 A192 | L198 L202 A134 L203 A135 A193 | L199 A132 L200 A133 L201 A193 | L204 L208 A138 L209 A139 A194 | L205 A136 L206 A137 L207 A194 | L210 L214 A142 L215 A143 A195 | L211 A140 L212 A141 L213 A195 | L216 L220 A146 L221 A147 A196 | L217 A144 L218 A145 L219 A196 | L222 L226 A150 L227 A151 A197 | L223 A148 L224 A149 L225 A197 | L228 L232 A154 L233 A155 A198 | L229 A152 L230 A153 L231 A198 | L234 L238 A158 L239 A159 A199 | L235 A156 L236 A157 L237 A199 bodies 34 2 33 27 22 24 25 23 37 19 36 41 38 31 18 40 32 26 30 29 28 15 6 14 16 35 8 5 9 10 11 17 3 39 21 7 13 20 4 12
sketch "Sketch4" plane through (0, 0, 6.7) normal (0, 0, 1) x (-1, 0, 0)
  line L0 (3.2654, 2.5) -> (101.4652, 2.5)
  line L1 (101.4652, 2.5) -> (101.4652, 6.7)
  line L2 (101.4652, 6.7) -> (3.2654, 6.7)
  line L3 (3.2654, 6.7) -> (3.2654, 2.5)
  arc A0 (-3.2654, -35.9157) -> (-0.3109, -33.4367) centre (-3.2654, -32.9157) ccw
  line L4 (-3.2654, -35.9157) -> (-101.4652, -35.9157)
  arc A1 (-104.4196, -33.4367) -> (-101.4652, -35.9157) centre (-101.4652, -32.9157) ccw
  line L5 (-104.4196, -33.4367) -> (-110.5811, 1.507)
  arc A2 (-108.1476, 4.9823) -> (-110.5811, 1.507) centre (-107.6267, 2.0279) ccw
  line L6 (-108.1476, 4.9823) -> (-61.1353, 13.2719)
  arc A3 (-60.6144, 13.3174) -> (-61.1353, 13.2719) centre (-60.6144, 10.3174) ccw
  line L7 (-60.6144, 13.3174) -> (-44.1162, 13.3174)
  arc A4 (-43.5952, 13.2719) -> (-44.1162, 13.3174) centre (-44.1162, 10.3174) ccw
  line L8 (-43.5952, 13.2719) -> (3.4171, 4.9823)
  arc A5 (5.8506, 1.507) -> (3.4171, 4.9823) centre (2.8961, 2.0279) ccw
  line L9 (5.8506, 1.507) -> (-0.3109, -33.4367)
  arc A6 (-2.0486, -37.6534) -> (0.9058, -35.1744) centre (-2.0486, -34.6534) ccw
  line L10 (0.9058, -35.1744) -> (7.5882, 2.7237)
  arc A7 (7.5882, 2.7237) -> (5.1548, 6.1991) centre (4.6338, 3.2446) ccw
  line L11 (5.1548, 6.1991) -> (-44.8119, 15.0095)
  arc A8 (-44.8119, 15.0095) -> (-45.3329, 15.0551) centre (-45.3329, 12.0551) ccw
  line L12 (-45.3329, 15.0551) -> (-59.3977, 15.0551)
  arc A9 (-59.3977, 15.0551) -> (-59.9186, 15.0095) centre (-59.3977, 12.0551) ccw
  line L13 (-59.9186, 15.0095) -> (-109.8853, 6.1991)
  arc A10 (-109.8853, 6.1991) -> (-112.3188, 2.7237) centre (-109.3644, 3.2446) ccw
  line L14 (-112.3188, 2.7237) -> (-105.6363, -35.1744)
  arc A11 (-105.6363, -35.1744) -> (-102.6819, -37.6534) centre (-102.6819, -34.6534) ccw
  line L15 (-102.6819, -37.6534) -> (-2.0486, -37.6534)
sketch "Sketch5" plane through (0, 0, 6.7) normal (0, 0, 1) x (-1, 0, 0)
  line L0 (-52.3653, -35.9157) -> (-58.3653, -35.9157)
  line L1 (-58.3653, -35.9157) -> (-58.3653, -37.6534)
  line L2 (-58.3653, -37.6534) -> (-52.3653, -37.6534)
  line L3 (-52.3653, -37.6534) -> (-52.3653, -35.9157)
  line L4 (-52.3653, -35.9157) -> (-46.3653, -35.9157)
  line L5 (-46.3653, -35.9157) -> (-46.3653, -37.6534)
  line L6 (-46.3653, -37.6534) -> (-52.3653, -37.6534)
  line L7 (-52.3653, -37.6534) -> (-52.3653, -35.9157)
  arc A0 (-3.2654, -35.9157) -> (-0.3109, -33.4367) centre (-3.2654, -32.9157) ccw
  line L8 (-3.2654, -35.9157) -> (-101.4652, -35.9157)
  arc A1 (-104.4196, -33.4367) -> (-101.4652, -35.9157) centre (-101.4652, -32.9157) ccw
  line L9 (-104.4196, -33.4367) -> (-110.5811, 1.507)
  arc A2 (-108.1476, 4.9823) -> (-110.5811, 1.507) centre (-107.6267, 2.0279) ccw
  line L10 (-108.1476, 4.9823) -> (-61.1353, 13.2719)
  arc A3 (-60.6144, 13.3174) -> (-61.1353, 13.2719) centre (-60.6144, 10.3174) ccw
  line L11 (-60.6144, 13.3174) -> (-44.1162, 13.3174)
  arc A4 (-43.5952, 13.2719) -> (-44.1162, 13.3174) centre (-44.1162, 10.3174) ccw
  line L12 (-43.5952, 13.2719) -> (3.4171, 4.9823)
  arc A5 (5.8506, 1.507) -> (3.4171, 4.9823) centre (2.8961, 2.0279) ccw
  line L13 (5.8506, 1.507) -> (-0.3109, -33.4367)
  arc A6 (-2.0486, -37.6534) -> (0.9058, -35.1744) centre (-2.0486, -34.6534) ccw
  line L14 (0.9058, -35.1744) -> (7.5882, 2.7237)
  arc A7 (7.5882, 2.7237) -> (5.1548, 6.1991) centre (4.6338, 3.2446) ccw
  line L15 (5.1548, 6.1991) -> (-44.8119, 15.0095)
  arc A8 (-44.8119, 15.0095) -> (-45.3329, 15.0551) centre (-45.3329, 12.0551) ccw
  line L16 (-45.3329, 15.0551) -> (-59.3977, 15.0551)
  arc A9 (-59.3977, 15.0551) -> (-59.9186, 15.0095) centre (-59.3977, 12.0551) ccw
  line L17 (-59.9186, 15.0095) -> (-109.8853, 6.1991)
  arc A10 (-109.8853, 6.1991) -> (-112.3188, 2.7237) centre (-109.3644, 3.2446) ccw
  line L18 (-112.3188, 2.7237) -> (-105.6363, -35.1744)
  arc A11 (-105.6363, -35.1744) -> (-102.6819, -37.6534) centre (-102.6819, -34.6534) ccw
  line L19 (-102.6819, -37.6534) -> (-2.0486, -37.6534)
  dimension "d35" = 6
  constraint horizontal L0
  constraint vertical L1
  constraint horizontal L2
  constraint vertical L3
  constraint horizontal L4
  constraint vertical L5
  constraint horizontal L6
  constraint vertical L7
  measures "d35" distance of L0.start L0.end
extrude "Extrude11" cut sketch "Sketch5" against normal blind 4.2 contours L0 L1 L2 L3 L7 L8 L19 | L3 L4 L5 L6 L7 L8 L19 bodies 1
fillet "Fillet1" radius 1.5 25 edges at (24.207, 37.6534, 6.7) (0.1203, 36.9516, 6.7) (-4.247, 16.2253, 6.7) (-7.0913, -4.9654, 6.7) (19.8286, -10.6043, 6.7) (45.0714, -15.0437, 6.7) (52.3653, -15.0551, 6.7) (59.6591, -15.0437, 6.7) (84.902, -10.6043, 6.7) (111.8218, -4.9654, 6.7) (108.9776, 16.2253, 6.7) (104.6103, 36.9516, 6.7) (80.5236, 37.6534, 6.7) (45.0714, -15.0437, 0) (19.8286, -10.6043, 0) (-7.0913, -4.9654, 0) (-4.247, 16.2253, 0) (0.1203, 36.9516, 0) (52.3653, 37.6534, 0) (104.6103, 36.9516, 0) (108.9776, 16.2253, 0) (111.8218, -4.9654, 0) (84.902, -10.6043, 0) (59.6591, -15.0437, 0) (52.3653, -15.0551, 0) on bodies 1
fillet "Fillet2" radius 1.2 40 edges at (88.2862, 16.7483, 4) (18.3093, 5.1637, 4) (91.7592, -2.9479, 4) (6.7248, -2.9479, 4) (81.9111, -4.6844, 4) (57.0055, 21.3869, 4) (29.8939, 13.2753, 4) (21.7823, 24.8599, 4) (2.0861, 28.3328, 4) (10.1977, 16.7483, 4) (96.3978, 28.3328, 4) (72.063, -6.4209, 4) (66.8536, 23.1234, 4) (86.5497, 26.5963, 4) (62.2149, -8.1573, 4) (-3.1233, -1.2114, 4) (38.0055, 1.6907, 4) (11.9342, 26.5963, 4) (76.7017, 24.8599, 4) (36.269, -8.1573, 4) (60.4785, 1.6907, 4) (8.4613, 6.9002, 4) (39.742, 11.5388, 4) (28.1574, 3.4272, 4) (78.4381, 15.0118, 4) (68.5901, 13.2753, 4) (101.6073, -1.2114, 4) (98.1343, 18.4847, 4) (90.0227, 6.9002, 4) (26.4209, -6.4209, 4) (70.3265, 3.4272, 4) (80.1746, 5.1637, 4) (99.8708, 8.6367, 4) (41.4785, 21.3869, 4) (0.3497, 18.4847, 4) (20.0458, 15.0118, 4) (16.5729, -4.6844, 4) (31.6304, 23.1234, 4) (58.742, 11.5388, 4) (-1.3868, 8.6367, 4) on bodies 2 3 4 5 6 7 8 9 10 11 12 13 14 15 16 17 18 19 20 21 22 23 24 25 26 27 28 29 30 31 32 33 34 35 36 37 38 39 40 41
fillet "Fillet3" radius 0.5 6 edges at (46.3653, 36.0346, 6.7) (46.3653, 37.2141, 6.2607) (46.3653, 37.6534, 3.85) (58.3653, 36.0346, 6.7) (58.3653, 37.2141, 6.2607) (58.3653, 37.6534, 3.85) on bodies 1
extrude "Extrude12" add sketch "Sketch1" along normal blind 1.5 contours A226 | A227 | A228 | A229 | A230 | A231 | A232 | A233 bodies 1
equation "plate_thickness = 2.5 mm"
equation "pole_height = 2.5 mm + plate_thickness + 0.1 mm" comment "reduced to 2.5mm (switch height)  + 0.1mm for tolerance. might be to low"
equation "wall_height = pole_height + pcb_thickness"
equation "pcb_thickness = 1.6 mm"
equation "d5 = plate_thickness"
equation "d7 = pole_height"
equation "d9 = wall_height"
equation "usb_cutout_length = 12 mm"
equation "key_base_thickness = 2 mm" comment "increased by 1"
equation "key_height = plate_thickness + 1.5 mm" comment "reduced by 1"
equation "d19 = key_rail_cutout_height"
equation "d21 = key_base_thickness"
equation "key_rail_cutout_height = ( plate_thickness ) - key_base_thickness"
equation "d24 = key_height"
equation "d35 = usb_cutout_length / 2"
equation "d36 = -wall_height + plate_thickness"
equation "case_walls_fillet = 1.5 mm"
equation "buttons_fillet = 1.2 mm"
equation "plate_thickness_screw_hole = plate_thickness - 1 mm"
equation "d55 = plate_thickness_screw_hole"
equation "d58 = case_walls_fillet"
equation "d60 = buttons_fillet"
